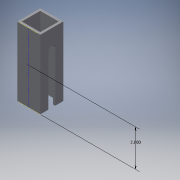
# Autodesk Inventor part: capForPost
Saved by Autodesk Inventor 2016 SP1 (Build 200210100, 210)
## iProperties
Created: 2016-02-08
Part Number: capForPost
Material: Generic
Document SubType Name: Modeling
Designer: steele
Density: 1 g/cm^3
Appearance: Default
Author: steele
Autodesk Inventor part; units mm, degrees
ref_plane "YZ Plane" through (0, 0, 0) normal (1, 0, 0) x (0, 1, 0)
ref_plane "XZ Plane" through (0, 0, 0) normal (0, 1, 0) x (-1, 0, 0)
ref_plane "XY Plane" through (0, 0, 0) normal (0, 0, 1) x (1, 0, 0)
sketch "Sketch1" plane through (0, 0, 0) normal (0, 1, 0) x (-1, 0, 0)
  line L0 (12.7, 12.7) -> (-12.7, 12.7)
  line L1 (-12.7, 12.7) -> (-12.7, -12.7)
  line L2 (-12.7, -12.7) -> (12.7, -12.7)
  line L3 (12.7, -12.7) -> (12.7, 12.7)
  line L4 (12.7, 12.7) -> (-12.7, -12.7) construction
  line L5 (-12.7, 12.7) -> (12.7, -12.7) construction
  line L6 (15.875, 15.875) -> (-15.875, 15.875)
  line L7 (-15.875, 15.875) -> (-15.875, -15.875)
  line L8 (-15.875, -15.875) -> (15.875, -15.875)
  line L9 (15.875, -15.875) -> (15.875, 15.875)
  line L10 (15.875, 15.875) -> (-15.875, -15.875) construction
  line L11 (-15.875, 15.875) -> (15.875, -15.875) construction
  point P0 (0, 0)
  dimension "d0" = 25.4
  dimension "d1" = 25.4
  dimension "d2" = 3.175
  dimension "d3" = 3.175
  constraints: 24 end point, 4 midpoint, 4 parallel, 2 horizontal, 2 perpendicular
  measures "d0" distance of L0.start L0.end
  measures "d1" distance of L2.end L0.start
  measures "d2" distance between parallel lines of L7 L1
  measures "d3" distance between parallel lines of L0 L6
extrude "Extrusion1" add sketch "Sketch1" along normal blind 95.1992
sketch "Sketch2" plane through (15.875, 0, 15.875) normal (1, 0, 0) x (0, 0, -1)
  line L0 (15.875, 0) -> (15.875, 69.7992) construction
  line L1 (20.6375, 0) -> (20.6375, 69.7992)
  line L2 (11.1125, 69.7992) -> (11.1125, 0)
  arc A0 (11.1125, 0) -> (20.6375, 0) centre (15.875, 0) ccw
  arc A1 (20.6375, 69.7992) -> (11.1125, 69.7992) centre (15.875, 69.7992) ccw
  line L3 (0, 0) -> (31.75, 0) projected
  point P0 (15.875, 34.8996)
  dimension "d6" = 4.7625
  dimension "d7" = 69.7992
  constraints: 8 end point, 4 point on circle, 4 tangent, 2 centre point, 1 midpoint, 1 parallel, 1 vertical
  measures "d6" radius of A1
  measures "d7" distance from line of L0.end L3
extrude "Extrusion2" cut sketch "Sketch2" against normal through all
sketch "Sketch3" plane through (-15.875, 0, 15.875) normal (0, 0, 1) x (1, 0, 0)
  line L0 (15.875, 0) -> (15.875, 95.1992) construction
  line L1 (28.575, 95.1992) -> (3.175, 95.1992) construction
  line L2 (0, 0) -> (31.75, 0) construction
  point P0 (15.875, 50.8)
  dimension "d10" = 50.8
  constraints: 2 end point, 1 midpoint, 1 point on line
  measures "d10" distance from line of point (15.875, 50.8) L2
body "Solid1"
